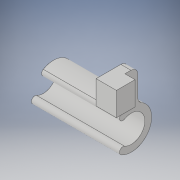
# Autodesk Inventor part: Roller_Spacer_P
Saved by Autodesk Inventor 2019 (Build 230136000, 136)
## iProperties
Created: 2019-10-12
Part Number: Roller_Spacer_P
Material: Generic
Document SubType Name: Modeling
Designer: James
Density: 1 g/cm^3
Appearance: Default
Author: James
Autodesk Inventor part; units mm, degrees
ref_plane "YZ Plane" through (0, 0, 0) normal (1, 0, 0) x (0, 1, 0)
ref_plane "XZ Plane" through (0, 0, 0) normal (0, 1, 0) x (-1, 0, 0)
ref_plane "XY Plane" through (0, 0, 0) normal (0, 0, 1) x (1, 0, 0)
sketch "Sketch1" plane through (0, 0, 0) normal (1, 0, 0) x (0, 1, 0)
  arc A0 (-3.4641, 2) -> (3.4641, 2) centre (0, 0) ccw
  arc A1 (-5.1962, 3) -> (5.1962, 3) centre (0, 0) ccw
  arc A2 (5.1962, 3) -> (3.4641, 2) centre (4.3301, 2.5) ccw
  arc A3 (-3.4641, 2) -> (-5.1962, 3) centre (-4.3301, 2.5) ccw
  dimension "d0" = 8
  dimension "d1" = 12
  dimension "d2" = 2.5
  constraints: 8 point on circle, 4 centre point, 4 tangent, 2 coincident, 1 horizontal alignment
  measures "d0" diameter of A0
  measures "d1" diameter of A1
  measures "d2" vertical distance of A2.centre point (0, 0)
extrude "Extrusion1" add sketch "Sketch1" against normal blind 26
sketch "Sketch2" plane through (0, 0, 0) normal (1, 0, 0) x (0, 0, -1)
  line L0 (-7.4, 15) -> (3.6, 15)
  line L1 (3.6, 15) -> (3.6, 4)
  line L2 (3.6, 4) -> (-7.4, 4)
  line L3 (-7.4, 4) -> (-7.4, 15)
  arc A0 (-2, -3.4641) -> (-2, 3.4641) centre (0, 0) ccw projected
  line L4 (-7.4, 15) -> (-1.9, 15)
  line L5 (-1.9, 15) -> (-1.9, 8)
  line L6 (-1.9, 8) -> (-7.4, 8)
  line L7 (-7.4, 8) -> (-7.4, 15)
  dimension "d5" = 11
  dimension "d6" = 11
  dimension "d7" = 7.4
  dimension "d8" = 5.5
  dimension "d9" = 7
  constraints: 16 end point, 4 parallel, 2 horizontal, 2 perpendicular, 1 tangent
  measures "d5" distance of L0.start L0.end
  measures "d6" distance of L0.end L1.end
  measures "d7" distance from line of point (0, 0) L3
  measures "d8" distance of L5.end L6.end
  measures "d9" distance of L4.end L5.end
extrude "Extrusion2" add sketch "Sketch2" along normal blind 3 contours L0 L5 L6 L3
sketch "Sketch3" plane through (0, 0, 0) normal (-1, 0, 0) x (0, 0, 1)
  line L0 (7.4, 15) -> (7.4, 8) projected
  line L1 (7.4, 15) -> (-1.9, 15)
  line L2 (1.9, 8) -> (7.4, 8)
  line L3 (7.4, 8) -> (7.4, 15)
  arc A0 (2, 3.4641) -> (2, -3.4641) centre (0, 0) ccw projected
  line L4 (7.4, 8) -> (1.9, 8) projected
  line L5 (1.9, 8) -> (1.9, 15) projected
  line L6 (1.9, 8) -> (1.9, 5.6912)
  arc A1 (3, 5.1962) -> (3, -5.1962) centre (0, 0) ccw projected
  line L7 (-1.9, 15) -> (-1.9, 5.6912)
  dimension "d12" = 1.9
  constraints: 10 end point, 2 point on circle, 2 vertical, 1 horizontal, 1 parallel, 1 point on line
  measures "d12" distance from line of point (0, 0) L7
extrude "Extrusion3" add sketch "Sketch3" along normal blind 3
fillet "Fillet1" radius 2 3 edges at (-1.5, 5.6912, 1.9) (-1.5, 5.6912, -1.9) (-1.5, 15, -1.9)
sketch "Sketch4" plane through (-26, 0, 0) normal (-1, 0, 0) x (0, 0, 1)
  line L0 (7.6885, 0) -> (-10.3871, 0)
  line L1 (-10.3871, 0) -> (-10.3871, 6.8992)
  line L2 (-10.3871, 6.8992) -> (7.6885, 6.8992)
  line L3 (7.6885, 6.8992) -> (7.6885, 0)
  point P0 (0, 0)
  constraints: 8 end point, 2 parallel, 1 horizontal, 1 perpendicular
extrude "Extrusion4" cut sketch "Sketch4" against normal blind 3
body "Solid1"
